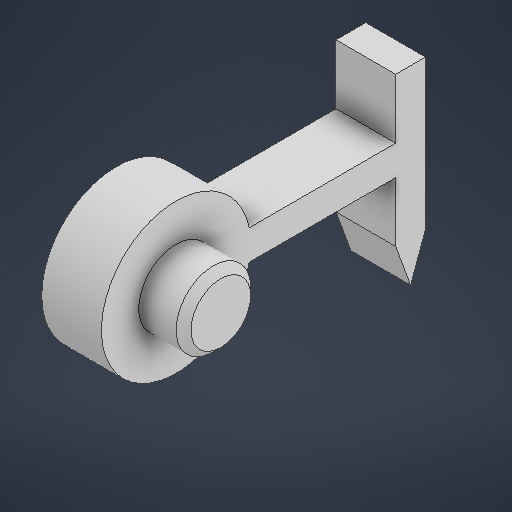
# Autodesk Inventor part: Peça4
Saved by Autodesk Inventor 2027 (Build 310192060, 192F)
## iProperties
Created: 2026-08-25
Part Number: Peça4
Material: Genérico
Document SubType Name: Modeling
Designer: guisg
Density: 1 g/cm^3
Appearance: Padrão
Author: guisg
Autodesk Inventor part; units mm, degrees
ref_plane "YZ Plane" through (0, 0, 0) normal (1, 0, 0) x (0, 1, 0)
ref_plane "XZ Plane" through (0, 0, 0) normal (0, 1, 0) x (-1, 0, 0)
ref_plane "XY Plane" through (0, 0, 0) normal (0, 0, 1) x (1, 0, 0)
sketch "Esboço1" plane through (0, 0, 0) normal (1, 0, 0) x (0, 1, 0)
  arc A0 (1, -4.9038) -> (-1, -4.9038) centre (0, 0) ccw
  line L0 (-1, -14.7248) -> (-1, -4.9038)
  line L1 (1, -14.72) -> (1, -4.9038)
  line L2 (1, -14.72) -> (5, -14.72)
  line L3 (5, -14.72) -> (5, -16.72)
  line L4 (5, -16.72) -> (-5, -16.72)
  line L5 (-1, -14.7248) -> (-4.9983, -14.7248)
  line L6 (-5, -16.72) -> (-7.74, -15.72)
  line L7 (-4.9983, -14.7248) -> (-7.74, -15.72)
  constraints: 16 end point, 2 horizontal, 2 perpendicular, 2 point on circle, 1 centre point, 1 parallel, 1 vertical
extrude "Extrusão1" add sketch "Esboço1" along normal blind 4
sketch "Esboço2" plane through (4, 0, 0) normal (1, 0, 0) x (0, 0, -1)
  circle A0 centre (0, 0) radius 2.5
  dimension "d20" = 5
  constraints: 1 centre point, 1 coincident
  measures "d20" diameter of A0
extrude "Extrusão2" add sketch "Esboço2" along normal blind 3
chamfer "Chanfro1" distance 0.5 angle 45 1 edges at (7, 0, 2.5) measured on face at (7, -0.6619, -1.2612)
